# Autodesk Inventor part: Zippy Flightmax 5000 6S 20C
Saved by Autodesk Inventor 2014 SP2 (Build 180246200, 246)
## iProperties
Created: 2014-05-19
Part Number: Zippy Flightmax 5000 6S 20C
Material: Generic
Document SubType Name: Modeling
Designer: dliu
Density: 1 g/cm^3
Appearance: Blue - Wall Paint - Glossy
Author: dliu
Autodesk Inventor part; units mm, degrees
ref_plane "YZ Plane" through (0, 0, 0) normal (1, 0, 0) x (0, 1, 0)
ref_plane "XZ Plane" through (0, 0, 0) normal (0, 1, 0) x (-1, 0, 0)
ref_plane "XY Plane" through (0, 0, 0) normal (0, 0, 1) x (1, 0, 0)
sketch "Sketch1" plane through (0, 0, 0) normal (0, 0, 1) x (1, 0, 0)
  line L0 (-26, 25) -> (26, 25)
  line L1 (26, 25) -> (26, -25)
  line L2 (26, -25) -> (-26, -25)
  line L3 (-26, -25) -> (-26, 25)
  line L4 (-26, 25) -> (26, -25) construction
  line L5 (26, 25) -> (-26, -25) construction
  point P0 (0, 0)
  dimension "d0" = 52
  dimension "d1" = 50
  constraints: 12 end point, 2 midpoint, 2 parallel, 1 horizontal, 1 perpendicular
  measures "d0" distance of L1.end L2.end
  measures "d1" distance of L0.end L1.end
extrude "Extrusion1" add sketch "Sketch1" along normal blind 142
body "Solid1"
